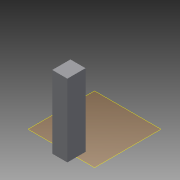
# Autodesk Inventor part: endstop_holder
Saved by Autodesk Inventor 2014 (Build 180170000, 170)
## iProperties
Created: 2014-02-17
Part Number: endstop_holder
Material: Generic
Document SubType Name: Modeling
Designer: stephen
Density: 1 g/cm^3
Appearance: Default
Author: stephen
Autodesk Inventor part; units mm, degrees
ref_plane "YZ Plane" through (0, 0, 0) normal (1, 0, 0) x (0, 1, 0)
ref_plane "XZ Plane" through (0, 0, 0) normal (0, 1, 0) x (-1, 0, 0)
ref_plane "XY Plane" through (0, 0, 0) normal (0, 0, 1) x (1, 0, 0)
ref_plane "Work Plane1" through (9.1076, 24.9687, 0) normal (0, 1, 0) x (1, 0, 0)
sketch "Sketch5" plane through (9.1076, 24.9687, 0) normal (0, 1, 0) x (1, 0, 0)
  line L0 (0, 0) -> (0, -14) projected
  line L1 (5, -14) -> (0, -14)
  line L2 (0, -14) -> (0, -7.9785)
  line L3 (0, -7.9785) -> (5, -7.9785)
  line L4 (5, -7.9785) -> (5, -14)
  point P0 (-9.1076, 0)
  constraints: 8 end point, 2 parallel, 1 horizontal, 1 perpendicular, 1 point on line
extrude "Extrusion5" add sketch "Sketch5" along normal blind 24
sketch "Sketch9" plane through (9.1076, 24.9687, 7.9785) normal (-1, 0, 0) x (0, 0, 1)
  line L0 (6.0215, 0) -> (6.0215, 24) projected
  line L1 (0, 24) -> (6.0215, 24) projected
  line L2 (1.981, 18) -> (1.981, 5.25) construction
  line L3 (0.856, 18) -> (0.856, 5.25)
  line L4 (3.106, 5.25) -> (3.106, 18)
  arc A0 (3.106, 18) -> (0.856, 18) centre (1.981, 18) ccw
  arc A1 (0.856, 5.25) -> (3.106, 5.25) centre (1.981, 5.25) ccw
  point P0 (-7.9785, -24.9687)
  point P1 (1.981, 11.625)
  dimension "d23" = 15
  dimension "d24" = 2.25
  dimension "d25" = 6
  dimension "d28" = 4.0405
  constraints: 8 end point, 4 point on circle, 4 tangent, 2 centre point, 2 parallel, 1 midpoint
  measures "d24" distance between parallel lines of L3 L4
  measures "d25" distance from line of L1 L2.start
  measures "d28" distance from line of L0 point (1.981, 11.625)
extrude "Extrusion9" cut sketch "Sketch9" against normal blind 25.4
body "Solid1"
